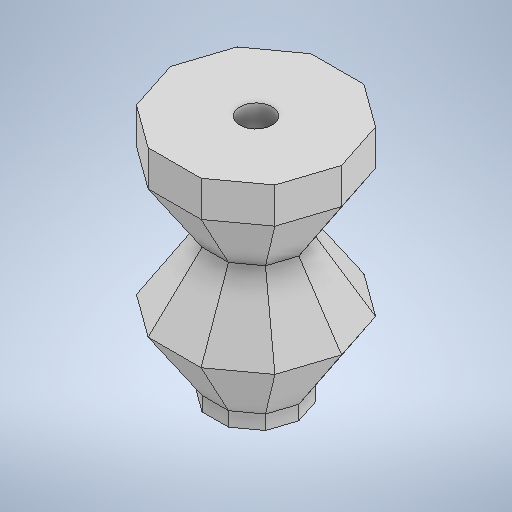
# Autodesk Inventor part: n_10
Saved by Autodesk Inventor 2025.1 (Build 291241000, 241)
## iProperties
Created: 2024-08-14
Part Number: n_10
Material: 일반
Document SubType Name: Modeling
Designer: 82103
Density: 1 g/cm^3
Appearance: 기본값
Author: 82103
Autodesk Inventor part; units mm, degrees
ref_plane "YZ Plane" through (0, 0, 0) normal (1, 0, 0) x (0, 1, 0)
ref_plane "XY Plane" through (0, 0, 0) normal (0, 0, 1) x (1, 0, 0)
sketch "스케치1" plane through (0, 0, 0) normal (0, 1, 0) x (-1, 0, 0)
  line L0 (9.7082, -7.0534) -> (3.7082, -11.4127)
  line L1 (3.7082, -11.4127) -> (-3.7082, -11.4127)
  line L2 (-3.7082, -11.4127) -> (-9.7082, -7.0534)
  line L3 (-9.7082, -7.0534) -> (-12, 0)
  line L4 (-12, 0) -> (-9.7082, 7.0534)
  line L5 (-9.7082, 7.0534) -> (-3.7082, 11.4127)
  line L6 (-3.7082, 11.4127) -> (3.7082, 11.4127)
  line L7 (3.7082, 11.4127) -> (9.7082, 7.0534)
  line L8 (9.7082, 7.0534) -> (12, 0)
  line L9 (12, 0) -> (9.7082, -7.0534)
  circle A0 centre (0, 0) radius 12 construction
  dimension "d0" = 24
  constraints: 20 end point, 2 coincident, 2 horizontal alignment, 23 other
ref_plane "작업 평면1" through (0, 9, 0) normal (0, 1, 0) x (-1, 0, 0)
sketch "스케치2" plane through (0, 9, 0) normal (0, 1, 0) x (-1, 0, 0)
  line L0 (4.8541, -3.5267) -> (1.8541, -5.7063)
  line L1 (1.8541, -5.7063) -> (-1.8541, -5.7063)
  line L2 (-1.8541, -5.7063) -> (-4.8541, -3.5267)
  line L3 (-4.8541, -3.5267) -> (-6, 0)
  line L4 (-6, 0) -> (-4.8541, 3.5267)
  line L5 (-4.8541, 3.5267) -> (-1.8541, 5.7063)
  line L6 (-1.8541, 5.7063) -> (1.8541, 5.7063)
  line L7 (1.8541, 5.7063) -> (4.8541, 3.5267)
  line L8 (4.8541, 3.5267) -> (6, 0)
  line L9 (6, 0) -> (4.8541, -3.5267)
  circle A0 centre (0, 0) radius 6 construction
  dimension "d2" = 12
  constraints: 20 end point, 2 coincident, 1 horizontal alignment, 24 other
loft "로프트1" add profiles "스케치2", "스케치1"
ref_plane "작업 평면2" through (0, 0, 0) normal (0, 1, 0) x (-1, 0, 0)
mirror "미러1" about plane through (0, 9, 0) normal (0, 1, 0) of "로프트1"
mirror "미러2" about plane through (0, 0, 0) normal (0, 1, 0) of "로프트1"
shell "쉘1" thickness 0.5 removed faces 0 ; own thickness 2 on faces at (-6.1492, -1.5, -8.4636) (-9.9496, -1.5, -3.2328) (-9.9496, -1.5, 3.2328) (-6.1492, -1.5, 8.4636) (0, -1.5, 10.4616) (6.1492, -1.5, 8.4636) (9.9496, -1.5, 3.2328) (9.9496, -1.5, -3.2328) (6.1492, -1.5, -8.4636) (0, -1.5, -10.4616) (0, 16.5, -10.4616) (6.1492, 16.5, -8.4636) (-6.1492, 16.5, -8.4636) (9.9496, 16.5, -3.2328) (9.9496, 16.5, 3.2328) (6.1492, 16.5, 8.4636) (0, 16.5, 10.4616) (-6.1492, 16.5, 8.4636) (-9.9496, 16.5, 3.2328) (-9.9496, 16.5, -3.2328)
sketch "스케치3" plane through (-1.8541, -9, -5.7063) normal (0, -1, 0) x (1, 0, 0)
  line L0 (-3, 2.1796) -> (0, 0) projected
  line L1 (0, 0) -> (3.7082, 0) projected
  line L2 (3.7082, 0) -> (6.7082, 2.1796) projected
  line L3 (6.7082, 2.1796) -> (7.8541, 5.7063) projected
  line L4 (7.8541, 5.7063) -> (6.7082, 9.2331) projected
  line L5 (6.7082, 9.2331) -> (3.7082, 11.4127) projected
  line L6 (3.7082, 11.4127) -> (0, 11.4127) projected
  line L7 (0, 11.4127) -> (-3, 9.2331) projected
  line L8 (-3, 9.2331) -> (-4.1459, 5.7063) projected
  line L9 (-4.1459, 5.7063) -> (-3, 2.1796) projected
  point P0 (1.8541, 5.7063)
extrude "돌출1" add sketch "스케치3" along normal blind 2
sketch "스케치4" plane through (-3.7082, 18, 11.4127) normal (0, 1, 0) x (1, 0, 0)
  line L0 (-6, 18.4661) -> (0, 22.8254) projected
  line L1 (-8.2918, 11.4127) -> (-6, 18.4661) projected
  line L2 (-6, 4.3593) -> (-8.2918, 11.4127) projected
  line L3 (0, 0) -> (-6, 4.3593) projected
  line L4 (7.4164, 0) -> (0, 0) projected
  line L5 (13.4164, 4.3593) -> (7.4164, 0) projected
  line L6 (15.7082, 11.4127) -> (13.4164, 4.3593) projected
  line L7 (13.4164, 18.4661) -> (15.7082, 11.4127) projected
  line L8 (7.4164, 22.8254) -> (13.4164, 18.4661) projected
  line L9 (0, 22.8254) -> (7.4164, 22.8254) projected
  point P0 (3.7082, 11.4127)
extrude "돌출2" add sketch "스케치4" along normal blind 5
sketch "스케치5" plane through (-3.7082, 23, 11.4127) normal (0, 1, 0) x (1, 0, 0)
  circle A0 centre (3.7082, 11.4127) radius 2.25
  dimension "d14" = 4.5
  constraints: 1 centre point, 1 coincident
  measures "d14" diameter of A0
extrude "돌출3" cut sketch "스케치5" against normal blind 6
